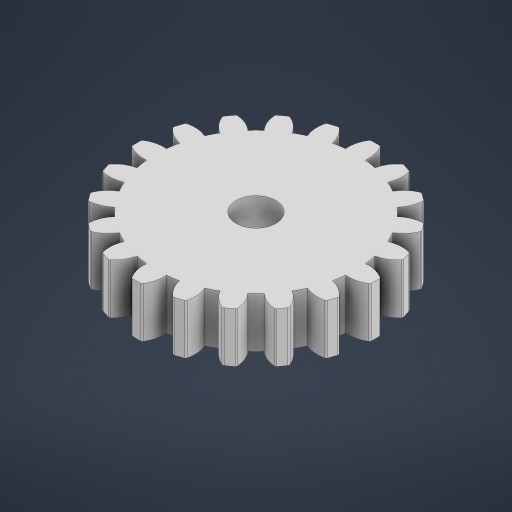
# Autodesk Inventor part: mid
Saved by Autodesk Inventor 2024 (Build 280153000, 153)
## iProperties
Created: 2023-05-10
Part Number: mid
Material: Типовые
Document SubType Name: Modeling
Designer: user
Density: 1 g/cm^3
Appearance: По умолчанию
Author: user
Autodesk Inventor part; units mm, degrees
ref_plane "YZ Plane" through (0, 0, 0) normal (1, 0, 0) x (0, 1, 0)
ref_plane "XZ Plane" through (0, 0, 0) normal (0, 1, 0) x (-1, 0, 0)
ref_plane "XY Plane" through (0, 0, 0) normal (0, 0, 1) x (1, 0, 0)
sketch "Эскиз1" plane through (0, 0, 0) normal (0, 0, 1) x (1, 0, 0)
  circle A0 centre (0, 0) radius 10
  circle A1 centre (0, 0) radius 2
  dimension "d0" = 20
  dimension "d20" = 4
  constraints: 2 centre point, 2 coincident
  measures "d0" diameter of A0
  measures "d20" diameter of A1
extrude "Выдавливание1" add sketch "Эскиз1" along normal blind 5
sketch "Эскиз2" plane through (0, 0, 5) normal (0, 0, 1) x (1, 0, 0)
  circle A0 centre (0, 0) radius 10 projected
  arc A1 (1, 9.9499) -> (-1, 9.9499) centre (0, 0) ccw
  arc A2 (-0.5, 11.9306) -> (-1, 9.9499) centre (1.985, 10.2499) ccw
  arc A3 (1, 9.9499) -> (0.5, 11.9306) centre (-1.985, 10.2499) ccw
  line L0 (0.5, 11.9306) -> (-0.5, 11.9306)
  point P0 (0, 11.9306)
  dimension "d9" = 1
  dimension "d10" = 2
  dimension "d11" = 3
  dimension "d12" = 3
  constraints: 8 point on circle, 3 centre point, 2 end point, 1 horizontal, 1 midpoint, 1 vertical alignment, 2 other
  measures "d9" distance of L0.start L0.end
  measures "d10" distance of A0.start A0.end
  measures "d11" radius of A3
  measures "d12" radius of A2
extrude "Выдавливание2" add sketch "Эскиз2" against normal up to surface (5 mm away) contours A0 A2 L0 A3
fillet "Сопряжение1" radius 0.2 2 edges at (-0.5, 11.9306, 2.5) (0.5, 11.9306, 2.5)
pattern_circular "Круговой массив1" count 20 over 360 about axis through (0, 0, 0) along (0, 0, 1) of "Сопряжение1", "Выдавливание2"
equation "\"d12\" = d11"
